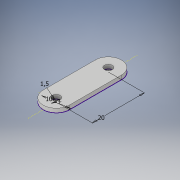
# Autodesk Inventor part: Mouth-Lever
Saved by Autodesk Inventor 2018.3 (Build 223284000, 284)
## iProperties
Created: 2018-05-18
Part Number: Mouth-Lever
Material: Generisch
Document SubType Name: Modeling
Designer: JochenAlt
Density: 1 g/cm^3
Appearance: Vorgabe
Author: JochenAlt
Autodesk Inventor part; units mm, degrees
ref_plane "YZ Plane" through (0, 0, 0) normal (1, 0, 0) x (0, 1, 0)
ref_plane "XZ Plane" through (0, 0, 0) normal (0, 1, 0) x (-1, 0, 0)
ref_plane "XY Plane" through (0, 0, 0) normal (0, 0, 1) x (1, 0, 0)
sketch "Skizze1" plane through (0, 0, 0) normal (0, 0, 1) x (1, 0, 0)
  line L0 (0, 31) -> (0, -11) construction
  line L1 (-7, 0) -> (7, 0) construction
  circle A0 centre (0, 0) radius 1.5
  arc A1 (-5, 0) -> (5, 0) centre (0, 0) ccw
  circle A2 centre (0, 20) radius 1.5
  arc A3 (5, 20) -> (-5, 20) centre (0, 20) ccw
  line L2 (-5, 20) -> (-5, 0)
  line L3 (5, 20) -> (5, 0)
  circle A4 centre (0, 0) radius 3
  circle A5 centre (0, 20) radius 3
  dimension "d0" = 3
  dimension "d1" = 10
  dimension "d4" = 1.5
  dimension "d7" = 20
  constraints: 6 centre point, 5 coincident, 4 end point, 4 point on circle, 3 equal radius, 2 tangent, 2 vertical, 1 point on line
  measures "d0" diameter of A0
  measures "d1" diameter of A1
  measures "d4" radial gap between concentric circles of A4 A0
  measures "d7" distance of point (0, 0) A2.centre
extrude "Extrusion1" add sketch "Skizze1" along normal blind 1.5 contours L2 A3 L3 A1 | A4 | A5
extrude "Extrusion2" add sketch "Skizze1" against normal blind 0.5 contours A4 | A5
